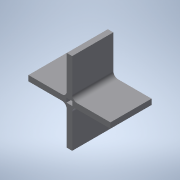
# Autodesk Inventor part: windmillv3
Saved by Autodesk Inventor 2022 (Build 260153000, 153)
## iProperties
Created: 2021-11-28
Part Number: windmillv3
Material: Generic
Document SubType Name: Modeling
Designer: haibo
Density: 1 g/cm^3
Appearance: Default
Author: haibo
Autodesk Inventor part; units mm, degrees
ref_plane "YZ Plane" through (0, 0, 0) normal (1, 0, 0) x (0, 1, 0)
ref_plane "XZ Plane" through (0, 0, 0) normal (0, 1, 0) x (-1, 0, 0)
ref_plane "XY Plane" through (0, 0, 0) normal (0, 0, 1) x (1, 0, 0)
sketch "Sketch1" plane through (0, 0, 0) normal (0, 0, 1) x (1, 0, 0)
  circle A0 centre (0, 0) radius 7.5
  dimension "d0" = 15
  constraints: 1 centre point, 1 coincident
  measures "d0" diameter of A0
extrude "Extrusion1" add sketch "Sketch1" along normal blind 10 and the other way blind 28.1
sketch "Sketch2" plane through (0, 0, 10) normal (0, 0, 1) x (1, 0, 0)
  line L0 (-2.7781, -1.9844) -> (2.7781, -1.9844)
  line L1 (2.7781, -1.9844) -> (2.7781, 1.9844)
  line L2 (2.7781, 1.9844) -> (-2.7781, 1.9844)
  line L3 (-2.7781, 1.9844) -> (-2.7781, -1.9844)
  line L4 (-2.7781, -1.9844) -> (2.7781, 1.9844) construction
  line L5 (2.7781, -1.9844) -> (-2.7781, 1.9844) construction
  point P0 (0, 0)
  dimension "d3" = 5.5563
  dimension "d4" = 3.9688
  constraints: 12 end point, 2 midpoint, 2 parallel, 1 horizontal, 1 perpendicular
  measures "d3" distance of L2.end L1.end
  measures "d4" distance of L1.end L0.end
extrude "Extrusion2" cut sketch "Sketch2" against normal blind 7.9375
ref_plane "Work Plane1" through (0, 0, 0) normal (0, 1, 0) x (0, 0, 1)
ref_plane "Work Plane2" through (0, 0, 0) normal (-1, 0, 0) x (0, 0, 1)
sketch "Sketch3" plane through (0, 0, 0) normal (0, 1, 0) x (0, 0, 1)
  point P0 (0, 0)
ref_plane "Work Plane3" through (0, 7.5, 0) normal (0, 1, 0) x (-1, 0, 0)
ref_plane "Work Plane4" through (0, -7.5, 0) normal (0, 1, 0) x (-1, 0, 0)
ref_plane "Work Plane5" through (-7.5, 0, 0) normal (-1, 0, 0) x (0, -1, 0)
ref_plane "Work Plane6" through (7.5, 0, 0) normal (-1, 0, 0) x (0, -1, 0)
sketch "Sketch4" plane through (0, 7.5, 0) normal (0, 1, 0) x (-1, 0, 0)
  point P0 (0, 0)
sketch "Sketch5" plane through (0, 7.5, 0) normal (0, 1, 0) x (-1, 0, 0)
  line L0 (7.5, 10) -> (-7.5, 10) projected
  line L1 (-2.5348, 10) -> (2.5348, 10)
  line L2 (2.5348, 10) -> (2.5348, -28.0998)
  line L3 (2.5348, -28.0998) -> (-2.5348, -28.0998)
  line L4 (-2.5348, -28.0998) -> (-2.5348, 10)
  point P0 (0, 0)
  constraints: 8 end point, 2 parallel, 2 point on line, 1 perpendicular
sketch "Sketch6" plane through (7.5, 0, 0) normal (-1, 0, 0) x (0, -1, 0)
  line L0 (-2.5348, 10) -> (2.5348, 10)
  line L1 (2.5348, 10) -> (2.5348, -28.0998)
  line L2 (2.5348, -28.0998) -> (-2.5348, -28.0998)
  line L3 (-2.5348, -28.0998) -> (-2.5348, 10)
  point P0 (0, 0)
  constraints: 8 end point, 2 parallel, 1 perpendicular
sketch "Sketch7" plane through (0, -7.5, 0) normal (0, 1, 0) x (-1, 0, 0)
  point P0 (0, 0)
sketch "Sketch8" plane through (0, -7.5, 0) normal (0, 1, 0) x (-1, 0, 0)
  line L0 (-2.5348, 10) -> (2.5348, 10)
  line L1 (2.5348, 10) -> (2.5348, -28.0998)
  line L2 (2.5348, -28.0998) -> (-2.5348, -28.0998)
  line L3 (-2.5348, -28.0998) -> (-2.5348, 10)
  point P0 (0, 0)
  constraints: 8 end point, 2 parallel, 1 perpendicular
sketch "Sketch9" plane through (0, -7.5, 0) normal (0, 1, 0) x (-1, 0, 0)
  point P0 (0, 0)
sketch "Sketch10" plane through (-7.5, 0, 0) normal (-1, 0, 0) x (0, -1, 0)
  line L0 (7.5, 10) -> (-7.5, 10) projected
  line L1 (-2.5422, 10) -> (2.5378, 10)
  line L2 (2.5378, 10) -> (2.5378, -28.1)
  line L3 (2.5378, -28.1) -> (-2.5422, -28.1)
  line L4 (-2.5422, -28.1) -> (-2.5422, 10)
  point P0 (0, 0)
  dimension "d9" = 5.08
  dimension "d10" = 38.1
  constraints: 8 end point, 2 parallel, 2 point on line, 1 perpendicular
  measures "d9" distance of L1.start L1.end
  measures "d10" distance of L1.end L2.end
extrude "Extrusion3" add sketch "Sketch5" along normal blind 30.48 and the other way blind 1.27
extrude "Extrusion4" add sketch "Sketch6" along normal blind 1.27 and the other way blind 30.48
extrude "Extrusion5" add sketch "Sketch10" along normal blind 30.48 and the other way blind 1.27
extrude "Extrusion6" add sketch "Sketch8" along normal blind 1.27 and the other way blind 30.48
sketch "Sketch11" plane through (0, 0, 10) normal (0, 0, 1) x (1, 0, 0)
  line L0 (2.5348, 7.0587) -> (2.5348, 6.9798)
  line L1 (37.98, 2.5348) -> (7.0587, 2.5348) projected
  line L2 (6.9798, 2.5348) -> (7.0587, 2.5348)
  arc A0 (2.5348, 6.9798) -> (6.9798, 2.5348) centre (6.9798, 6.9798) ccw
  arc A1 (7.0587, 2.5348) -> (2.5348, 7.0587) centre (0, 0) ccw projected
  arc A2 (7.0587, 2.5348) -> (2.5348, 7.0587) centre (0, 0) ccw
  arc A3 (-2.5348, 7.0587) -> (-7.0587, 2.5348) centre (0, 0) ccw
  arc A4 (-6.9798, 2.5348) -> (-2.5348, 6.9798) centre (-6.9798, 6.9798) ccw
  line L3 (-7.0587, 2.5348) -> (-6.9798, 2.5348)
  line L4 (-2.5348, 6.9798) -> (-2.5348, 7.0587)
  arc A5 (-7.0587, -2.5348) -> (-2.5348, -7.0587) centre (0, 0) ccw
  arc A6 (-2.5348, -6.9798) -> (-6.9798, -2.5348) centre (-6.9798, -6.9798) ccw
  line L5 (-2.5348, -7.0587) -> (-2.5348, -6.9798)
  line L6 (-6.9798, -2.5348) -> (-7.0587, -2.5348)
  arc A7 (2.5348, -7.0587) -> (7.0587, -2.5348) centre (0, 0) ccw
  arc A8 (6.9798, -2.5348) -> (2.5348, -6.9798) centre (6.9798, -6.9798) ccw
  line L7 (7.0587, -2.5348) -> (6.9798, -2.5348)
  line L8 (2.5348, -6.9798) -> (2.5348, -7.0587)
  dimension "d29" = 4.445
  dimension "d32" = 360
  constraints: 16 end point, 16 point on circle, 8 centre point, 2 perpendicular, 2 tangent, 1 concentric, 41 other
  measures "d29" radius of A0
extrude "Extrusion7" cut sketch "Sketch11" against normal blind 38.1
body "Solid1"
